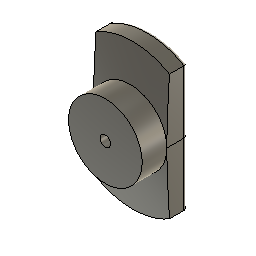
loquet_placard_WC v4 (Autodesk Fusion 360 design; units mm, degrees)
Autodesk Fusion 360 part; units mm, degrees
note: some values were not read from the file. Chosen so that the rebuilt part matches the saved one: which pieces of a blend or face edit are solid.
sketch "Esquisse1" plane through (0, 0, 0) normal (0, 1, 0) x (1, 0, 0)
  circle A0 centre (0, 0) radius 42.5
  dimension "d1" = 85
  constraint coincident A0.centre origin
  measures "d1" diameter of A0
extrude "Extrusion1" add sketch "Esquisse1" along normal blind 12
sketch "Esquisse2" plane through (0, 0, 0) normal (0, -1, 0) x (1, 0, 0)
  circle A0 centre (0, 0) radius 42.5
  circle A1 centre (0, 0) radius 21.5
  dimension "d4" = 43
  constraint coincident A0.centre A1.centre
  measures "d4" diameter of A1
extrude "Extrusion2" add sketch "Esquisse2" along normal blind 14.5 contours A1
sketch "Esquisse3" plane through (0, -14.5, 0) normal (0, -1, 0) x (1, 0, 0)
  circle A0 centre (0, 0) radius 21.5
  circle A1 centre (0, 0) radius 3.1
  dimension "d7" = 6.2
  constraint coincident A0.centre A1.centre
  measures "d7" diameter of A1
extrude "Extrusion3" cut sketch "Esquisse3" against normal blind 30 contours A1
chamfer "Chanfrein1" distance 1.5 distance2 21 1 edges at (-39.6239, 0, 15.3687) measured on face at (42.4472, 8, 2.1185)
sketch "Esquisse4" plane through (0, 0, 0) normal (0, -1, 0) x (1, 0, 0)
  circle A0 centre (0, 0) radius 42.5
  circle A1 centre (0, 0) radius 42.5
  line L0 (-21.5, 0) -> (-21.4682, 36.6792)
  line L1 (-21.5, 0) -> (-21.472, -36.677)
  line L2 (21.5, 36.6606) -> (21.5, 0)
  line L3 (21.5, 0) -> (21.5109, -36.6542)
  constraint coincident A0 L0.end
  constraint coincident A1 L0.end
  constraint coincident A1 L1.end
  constraint coincident A0 L2.start
  constraint coincident A0 L3.end
extrude "Extrusion4" cut sketch "Esquisse4" against normal blind 30 contours A0 A1 L2 L3 | A0 A1 L0 L1
sketch "Esquisse5" plane through (0, 12, 0) normal (0, 1, 0) x (-1, 0, 0)
  circle A0 centre (0, 0) radius 3.1
  line L0 (-21.5, 36.6606) -> (-21.5, 0)
  line L1 (-21.5, 0) -> (-21.5109, -36.6542)
  arc A1 (-21.5109, -36.6542) -> (21.472, -36.677) centre (0, 0) ccw
  line L2 (21.472, -36.677) -> (21.5, 0)
  line L3 (21.5, 0) -> (21.4682, 36.6792)
  arc A2 (21.4682, 36.6792) -> (-21.5, 36.6606) centre (0, 0) ccw
  circle A3 centre (0, 0) radius 9.1
  dimension "d18" = 18.2
  constraint coincident A0.centre A1.centre
  measures "d18" diameter of A3
extrude "Extrusion5" cut sketch "Esquisse5" against normal blind 7 contours A3
fillet "Congé1" radius 2 6 edges at (21.5, 12, 18.3303) (21.5055, 12, -18.3271) (0.0226, 12, -42.5) (-21.486, 12, -18.3385) (-21.4841, 12, 18.3396) (0.0184, 12, 42.5)
